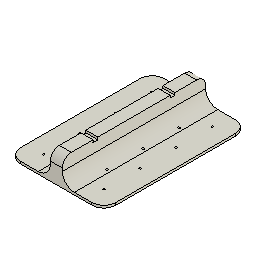
Tempeh-mould-lid-8x12-lid (Autodesk Fusion 360 design; units mm, degrees)
Autodesk Fusion 360 part; units mm, degrees
note: some values were not read from the file. Set by a fixed rule: which sketch regions a step uses.
sketch "Sketch-footprint-box" plane through (0, 0, 0) normal (0, 0, 1) x (1, 0, 0)
  line L0 (-40, 60) -> (40, 60) construction
  line L1 (40, 60) -> (40, -60) construction
  line L2 (40, -60) -> (-40, -60) construction
  line L3 (-40, -60) -> (-40, 60) construction
  line L4 (-40, 60) -> (40, -60) construction
  line L5 (40, 60) -> (-40, -60) construction
  line L6 (39.5, 59.5) -> (-39.5, 59.5)
  line L7 (-39.5, 59.5) -> (-39.5, -59.5)
  line L8 (-39.5, -59.5) -> (39.5, -59.5)
  line L9 (39.5, -59.5) -> (39.5, 59.5)
  line L10 (39.5, 59.5) -> (-39.5, -59.5) construction
  line L11 (-39.5, 59.5) -> (39.5, -59.5) construction
  dimension "width" = 80
  dimension "length" = 120
  dimension "d104" = 0.5
  dimension "d105" = 0.5
  constraint horizontal L0
  constraint vertical L1
  constraint horizontal L2
  constraint vertical L3
  constraint midpoint L5 origin
  constraint horizontal L6
  constraint perpendicular L6 L7
  constraint parallel L6 L8
  constraint parallel L7 L9
  constraint coincident L10 origin
  constraint coincident L11 origin
  measures "width" distance of L0.start L0.end
  measures "length" distance of L0.start L2.end
  measures "d104" distance of L0 L6
  measures "d105" distance of L3 L7
extrude "Extrude1" add sketch "Sketch-footprint-box" along normal blind 2
sketch "Sketch-lid" plane through (0, 0, 2) normal (0, 0, 1) x (-1, 0, 0)
  line L0 (5, -59.5) -> (-5, -59.5)
  line L1 (-5, -59.5) -> (-5, 59.5)
  line L2 (-5, 59.5) -> (5, 59.5)
  line L3 (5, 59.5) -> (5, -59.5)
  line L4 (5, -59.5) -> (-5, 59.5) construction
  line L5 (-5, -59.5) -> (5, 59.5) construction
  line L6 (-39.5, 59.5) -> (-39.5, -59.5)
  line L7 (-39.5, -59.5) -> (39.5, -59.5)
  line L8 (39.5, -59.5) -> (39.5, 59.5)
  line L9 (39.5, 59.5) -> (-39.5, 59.5)
  dimension "handle_width" = 10
  constraint horizontal L0
  constraint vertical L1
  constraint horizontal L2
  constraint vertical L3
  constraint midpoint L5 origin
  constraint coincident L1.end L9
  measures "handle_width" distance of L0.start L0.end
extrude "Extrude2" add sketch "Sketch-lid" along normal blind 20 contours L0 L1 L2 L3 L7 L9
extrude "Extrude8" add 1 faces at (-13.1667, 19.8333, 0) along direction (0, 0, -1) blind 0.0001
draft "Draft18" angle 0 neutral plane through (0, 0, 22) pull (0, 0, 1) 1 faces at (-5, -19.8333, 8.6667)
draft "Draft19" angle 0 neutral plane through (0, 0, 22) pull (0, 0, 1) 1 faces at (5, 19.8333, 15.3333)
draft "Draft20" angle 0 neutral plane through (0, 0, 22) pull (0, 0, 1) 1 faces at (-1.6667, -59.5, 15.3333)
draft "Draft21" angle 0 neutral plane through (0, 0, 22) pull (0, 0, 1) 1 faces at (1.6667, 59.5, 15.3333)
draft "Draft22" angle 0 neutral plane through (0, 0, 2) pull (0, 0, 1) 1 faces at (39.5, 19.8333, 0.6666)
draft "Draft23" angle 0 neutral plane through (0, 0, 2) pull (0, 0, 1) 1 faces at (-39.5, 19.8333, 1.3333)
fillet "Fillet5" radius 10 4 edges at (39.5, -59.5, 0.9999) (39.5, 59.5, 1) (-39.5, 59.5, 1) (-39.5, -59.5, 1)
fillet "Fillet6" radius 10 2 edges at (-5, 0, 2) (5, 0, 2)
fillet "Fillet7" radius 7.5 2 edges at (0, -59.5, 22) (0, 59.5, 22)
sketch "Sketch-notches-handle" plane through (0, 0, 22) normal (0, 0, 1) x (-1, 0, 0)
  line L0 (5, -52) -> (5, 52)
  line L1 (-5, 52) -> (-5, -52)
  line L2 (5, -34) -> (-5, -34)
  line L3 (-5, -34) -> (-5, -30)
  line L4 (-5, -30) -> (5, -30)
  line L5 (5, -30) -> (5, -34)
  line L6 (5, 30) -> (-5, 30)
  line L7 (-5, 30) -> (-5, 34)
  line L8 (-5, 34) -> (5, 34)
  line L9 (5, 34) -> (5, 30)
  line L10 (5, -30) -> (-5, 30) construction
  line L11 (-5, -30) -> (5, 30) construction
  line L12 (5, -30) -> (-5, -34) construction
  line L13 (5, -34) -> (-5, -30) construction
  line L14 (5, 34) -> (-5, 30) construction
  line L15 (-5, 34) -> (5, 30) construction
  circle A0 centre (0, -32) radius 0.75
  circle A1 centre (0, 32) radius 0.75
  line L16 (0, -30) -> (0, 0) construction
  line L17 (0, 0) -> (0, 30) construction
  line L18 (-5, -52) -> (5, -52)
  line L19 (5, 52) -> (-5, 52)
  dimension "handle_pocket" = 4
  dimension "d29" = 4
  dimension "hole_diameter" = 1.5
  dimension "d48" = 1.5
  dimension "d79" = 60
  constraint horizontal L2
  constraint vertical L3
  constraint horizontal L4
  constraint vertical L5
  constraint coincident L1 L3.end
  constraint coincident L0 L2.start
  constraint horizontal L6
  constraint vertical L7
  constraint horizontal L8
  constraint vertical L9
  constraint coincident L1 L7.end
  constraint coincident L0 L6.start
  constraint midpoint L10 L16.end
  constraint coincident L16.end L17.start
  constraint midpoint L13 A0.centre
  constraint midpoint L15 A1.centre
  constraint midpoint L4 L16.start
  constraint midpoint L6 L17.end
  measures "handle_pocket" distance of L2.start L4.end
  measures "d29" distance of L6.start L8.end
  measures "hole_diameter" diameter of A0
  measures "d48" diameter of A1
  measures "d79" distance of L3.end L6.end
extrude "Extrude3" cut sketch "Sketch-notches-handle" against normal blind 2 contours L0 L1 L2 L3 L4 L5 | L0 L1 L6 L7 L8 L9 | A0 | A1
sketch "Sketch-holes" plane through (0, 0, 2) normal (0, 0, 1) x (-1, 0, 0)
  line L0 (-40, -60) -> (40, -60) construction
  line L1 (40, -60) -> (40, 60) construction
  line L2 (40, 60) -> (-40, 60) construction
  line L3 (-40, 60) -> (-40, -60) construction
  line L4 (-40, -60) -> (40, 60) construction
  line L5 (40, -60) -> (-40, 60) construction
  line L6 (-25, -45) -> (25, -45) construction
  line L7 (25, -45) -> (25, 45) construction
  line L8 (25, 45) -> (-25, 45) construction
  line L9 (-25, 45) -> (-25, -45) construction
  circle A0 centre (25, -45) radius 0.75
  circle A1 centre (12.5, -30) radius 0.75
  circle A2 centre (12.5, 0) radius 0.75
  circle A3 centre (0, 30) radius 0.75
  circle A4 centre (25, 45) radius 0.75
  line L10 (15, -59.5) -> (29.5, -59.5)
  line L11 (39.5, -49.5) -> (39.5, 49.5)
  line L12 (29.5, 59.5) -> (15, 59.5)
  line L13 (-39.5, 49.5) -> (-39.5, -49.5)
  line L14 (15, 59.5) -> (15, -59.5)
  line L15 (-15, -59.5) -> (-15, 59.5)
  line L16 (-15, 59.5) -> (-29.5, 59.5)
  line L17 (-29.5, -59.5) -> (-15, -59.5)
  circle A5 centre (-12.5, -30) radius 0.75
  circle A6 centre (-25, -15) radius 0.75
  circle A7 centre (-25, 15) radius 0.75
  circle A8 centre (-12.5, 30) radius 0.75
  circle A9 centre (-25, 45) radius 0.75
  circle A10 centre (25, -15) radius 0.75
  circle A11 centre (-12.5, 0) radius 0.75
  circle A12 centre (25, 15) radius 0.75
  circle A13 centre (12.5, 30) radius 0.75
  circle A14 centre (-25, -45) radius 0.75
  circle A15 centre (0, -30) radius 0.75
  arc A16 (-29.5, 59.5) -> (-39.5, 49.5) centre (-29.5, 49.5) ccw
  arc A17 (-39.5, -49.5) -> (-29.5, -59.5) centre (-29.5, -49.5) ccw
  arc A18 (29.5, -59.5) -> (39.5, -49.5) centre (29.5, -49.5) ccw
  arc A19 (39.5, 49.5) -> (29.5, 59.5) centre (29.5, 49.5) ccw
  dimension "d52" = 80
  dimension "d53" = 120
  dimension "hole_offset" = -15
  dimension "d55" = 1.5
  dimension "width_holes_surface" = -50
  dimension "length_holes_surface" = 90
  constraint horizontal L0
  constraint perpendicular L0 L1
  constraint parallel L0 L2
  constraint parallel L1 L3
  constraint coincident L4 origin
  constraint coincident L5 origin
  constraint coincident L6.end L7.start
  measures "d52" distance of L1.end L2.end
  measures "d53" distance of L0.end L1.end
  measures "d55" diameter of A0
extrude "Extrude7" cut sketch "Sketch-holes" along normal mid plane 36 contours A0 | A1 | A2 | A4 | A5 | A6 | A7 | A8 | A9 | A10 | A11 | A12 | A13 | A14
equation "thickness = 2 mm"
equation "handle_heigth = 20 mm"
equation "draft = 0 deg"
equation "corner_fillet = 10.00 mm"
equation "handle_end_fillet = 7.5 mm"
equation "handle_base_fillet = 10 mm"
equation "d29 = handle_pocket"
equation "handle_pocket_depth = -2.00 mm"
equation "mini_fillet = 1 mm"
equation "d48 = hole_diameter"
equation "hole_depth = -37.00 mm"
equation "d52 = width"
equation "d53 = length"
equation "d55 = hole_diameter"
equation "width_holes_number = 5" comment "width / 20 +1"
equation "length_holes_number = 7" comment "length / 20 + 1"
equation "width_holes_surface = -width - 2 * hole_offset"
equation "length_holes_surface = length + 2 * hole_offset"
equation "extra_bottom_thickness = 0.0001 mm"
equation "d79 = length / 2"
equation "width_offset = 0.5 mm"
equation "length_offset = 0.5 mm"
equation "d84 = draft"
equation "d86 = draft"
equation "d88 = draft"
equation "d90 = draft"
equation "d92 = draft"
equation "d94 = draft"
equation "d97 = corner_fillet"
equation "d99 = handle_base_fillet"
equation "d101 = handle_end_fillet"
equation "d104 = width_offset"
equation "d105 = length_offset"
named bodies: "lid"
